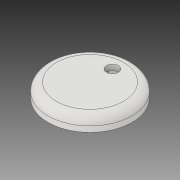
# Autodesk Inventor part: base
Saved by Autodesk Inventor 2019 (Build 230136000, 136)
## iProperties
Created: 2019-01-04
Part Number: base
Material: PC/ABS Plastic
Document SubType Name: Modeling
Designer: Callum Snowden
Mass: 9.20493 g
Surface Area: 73.0399 cm^2
Volume: 25.7644 cm^3
Density: 0.357273 g/cm^3
Appearance: Smooth - White
Author: Callum Snowden
## iProperties of the stored document base_3DPrint.ipt
Created: 2019-01-04
Part Number: base_3DPrint
Material: Generic
Document SubType Name: Modeling
Designer: Callum Snowden
Mass: 25.7644 g
Surface Area: 73.0399 cm^2
Volume: 25.7644 cm^3
Density: 1 g/cm^3
Appearance: Default
Author: Callum Snowden
Autodesk Inventor part; units mm, degrees
ref_plane "YZ Plane" through (0, 0, 0) normal (1, 0, 0) x (0, 1, 0)
ref_plane "XZ Plane" through (0, 0, 0) normal (0, 1, 0) x (-1, 0, 0)
ref_plane "XY Plane" through (0, 0, 0) normal (0, 0, 1) x (1, 0, 0)
sketch "Sketch1" plane through (0, 0, 0) normal (0, 1, 0) x (-1, 0, 0)
  circle A0 centre (0, 0) radius 30
  circle A1 centre (0, -16) radius 4.25
  dimension "d0" = 60
  dimension "d1" = 8.5
  dimension "d2" = 16
  constraints: 2 centre point, 1 coincident
  measures "d0" diameter of A0
  measures "d1" diameter of A1
  measures "d2" distance of point (0, 0) A1.centre
extrude "Extrusion1" add sketch "Sketch1" along normal blind 10
sketch "Sketch2" plane through (0, 0, 0) normal (0, -1, 0) x (1, 0, 0)
  circle A0 centre (0, -16) radius 4.25 construction
  line L0 (6.55, -19.7816) -> (0, -23.5633)
  line L1 (0, -23.5633) -> (-6.55, -19.7816)
  line L2 (-6.55, -19.7816) -> (-6.55, -12.2184)
  line L3 (-6.55, -12.2184) -> (0, -8.4367)
  line L4 (0, -8.4367) -> (6.55, -12.2184)
  line L5 (6.55, -12.2184) -> (6.55, -19.7816)
  point P0 (0, 0)
  dimension "d5" = 13.1
  constraints: 12 end point, 1 coincident, 13 other
  measures "d5" distance between parallel lines of L2 L5
extrude "Extrusion2" cut sketch "Sketch2" against normal blind 6
fillet "Fillet1" radius 6 1 edges at (30, 10, 0)
body "Solid1"
